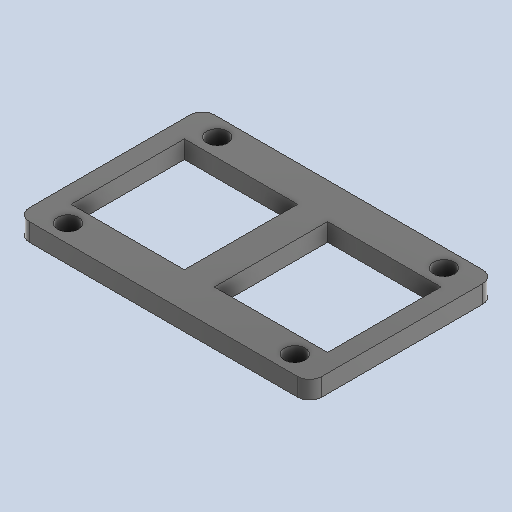
# Autodesk Inventor part: StartStopSwitch_upper_cover
Saved by Autodesk Inventor 2022.4 (Build 264492000, 492)
## iProperties
Created: 2021-10-05
Part Number: StartStopSwitch_upper_cover
Material: アセタール樹脂、黒
Document SubType Name: Modeling
Designer: Masato Kubotera
Density: 1.425 g/cm^3
Appearance: 滑らか - 黒
Description: PLA
Mass: 3.22797 g
Surface Area: 25.6781 cm^2
Volume: 2.26525 cm^3
Author: Masato Kubotera
Autodesk Inventor part; units mm, degrees
ref_plane "YZ Plane" through (0, 0, 0) normal (1, 0, 0) x (0, 1, 0)
ref_plane "XZ Plane" through (0, 0, 0) normal (0, 1, 0) x (-1, 0, 0)
ref_plane "XY Plane" through (0, 0, 0) normal (0, 0, 1) x (1, 0, 0)
derived "Switch_basis.ipt"
sketch "スケッチ1" plane through (0, 0, 0) normal (0, 0, 1) x (1, 0, 0)
  line L0 (23, 12.5) -> (23, -12.5) construction
  line L1 (23, 12.5) -> (-23, -12.5) construction
  circle A0 centre (-19, 12.5) radius 3 construction
  line L2 (-3, -9) -> (-21, -9) construction
  line L3 (-21, -9) -> (-21, 9) construction
  line L4 (-21, 9) -> (-3, 9) construction
  line L5 (-3, 9) -> (-3, -9) construction
  line L6 (-3, -9) -> (-21, 9) construction
  line L7 (-21, -9) -> (-3, 9) construction
  line L8 (-23, 0) -> (23, 0) construction
  line L9 (0, 12.5) -> (0, -12.5) construction
  line L10 (3, -9) -> (21, -9) construction
  line L11 (21, -9) -> (21, 9) construction
  line L12 (3, 9) -> (3, -9) construction
  line L13 (21, 9) -> (3, 9) construction
  line L14 (3, -9) -> (21, 9) construction
  line L15 (21, -9) -> (3, 9) construction
  line L16 (-23, 12.5) -> (23, -12.5) construction
  line L17 (-23, 12.5) -> (-20.6, 12.5) construction
  arc A1 (-20.6, 12.5) -> (-17.4, 12.5) centre (-19, 12.5) ccw construction
  arc A2 (-17.4, -12.5) -> (-20.6, -12.5) centre (-19, -12.5) ccw construction
  line L18 (-23, -12.5) -> (-20.6, -12.5) construction
  arc A3 (17.4, 12.5) -> (20.6, 12.5) centre (19, 12.5) ccw construction
  line L19 (23, 12.5) -> (20.6, 12.5) construction
  line L20 (23, -12.5) -> (20.6, -12.5) construction
  arc A4 (20.6, -12.5) -> (17.4, -12.5) centre (19, -12.5) ccw construction
  line L21 (-17.4, 12.5) -> (17.4, 12.5) construction
  line L22 (17.4, -12.5) -> (-17.4, -12.5) construction
  line L23 (-23, 12.5) -> (-23, -12.5) construction
  line L24 (-24.5, 15.5) -> (24.5, 15.5)
  line L25 (24.5, 15.5) -> (24.5, -15.5)
  line L26 (24.5, -15.5) -> (-24.5, -15.5)
  line L27 (-24.5, -15.5) -> (-24.5, 15.5)
  line L28 (-24.5, 15.5) -> (24.5, -15.5) construction
  line L29 (24.5, 15.5) -> (-24.5, -15.5) construction
  line L30 (-23.25, 12.75) -> (23.25, 12.75) construction
  line L31 (23.25, 12.75) -> (23.25, -12.75) construction
  line L32 (23.25, -12.75) -> (-23.25, -12.75) construction
  line L33 (-23.25, -12.75) -> (-23.25, 12.75) construction
  line L34 (-23.25, 12.75) -> (23.25, -12.75) construction
  line L35 (23.25, 12.75) -> (-23.25, -12.75) construction
  circle A5 centre (19, 12.5) radius 3 construction
  circle A6 centre (-19, -12.5) radius 3 construction
  circle A7 centre (19, -12.5) radius 3 construction
  line L36 (-21.5, 9.5) -> (-2.5, 9.5)
  line L37 (-2.5, 9.5) -> (-2.5, -9.5)
  line L38 (-2.5, -9.5) -> (-21.5, -9.5)
  line L39 (-21.5, -9.5) -> (-21.5, 9.5)
  line L40 (-21.5, 9.5) -> (-2.5, -9.5) construction
  line L41 (-2.5, 9.5) -> (-21.5, -9.5) construction
  line L42 (21.5, 9.5) -> (2.5, 9.5)
  line L43 (2.5, 9.5) -> (2.5, -9.5)
  line L44 (2.5, -9.5) -> (21.5, -9.5)
  line L45 (21.5, -9.5) -> (21.5, 9.5)
  circle A8 centre (-19, 12.5) radius 1.75
  circle A9 centre (19, 12.5) radius 1.75
  circle A10 centre (-19, -12.5) radius 1.75
  circle A11 centre (19, -12.5) radius 1.75
  point P0 (0, 0)
  point P1 (-12, 0)
  point P2 (12, 0)
  point P3 (-12, 0)
  point P4 (0, 0)
  point P5 (0, 0)
  dimension "d2" = 0.5
  dimension "d3" = 3.5
  measures "d2" distance between parallel lines of L36 L4
  measures "d3" diameter of A8
extrude "押し出し1" add sketch "スケッチ1" along normal blind 3
fillet "フィレット1" radius 2 4 edges at (-24.5, 15.5, 1.5) (-24.5, -15.5, 1.5) (24.5, -15.5, 1.5) (24.5, 15.5, 1.5)
